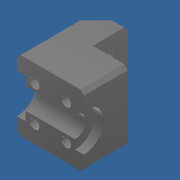
# Autodesk Inventor part: Print_Parts_L
Saved by Autodesk Inventor 2020 (Build 240168000, 168)
## iProperties
Created: 2020-10-05
Part Number: Print_Parts_L
Material: PC/ABS プラスチック
Document SubType Name: Modeling
Designer: kenta iguchi
Density: 0.357273 g/cm^3
Appearance: 滑らか - 黒
Author: kenta iguchi
Autodesk Inventor part; units mm, degrees
ref_plane "YZ Plane" through (0, 0, 0) normal (1, 0, 0) x (0, 1, 0)
ref_plane "XZ Plane" through (0, 0, 0) normal (0, 1, 0) x (-1, 0, 0)
ref_plane "XY Plane" through (0, 0, 0) normal (0, 0, 1) x (1, 0, 0)
sketch "スケッチ1" plane through (0, 0, 0) normal (0, 0, 1) x (1, 0, 0)
  line L0 (-10, -20) -> (10, -20)
  line L1 (10, -20) -> (10, 20)
  line L2 (10, 20) -> (-10, 20)
  line L3 (-10, 20) -> (-10, -20)
  line L4 (-10, -20) -> (10, 20) construction
  line L5 (10, -20) -> (-10, 20) construction
  point P0 (0, 0)
  dimension "d0" = 20
  dimension "d1" = 40
  constraints: 12 end point, 2 midpoint, 2 parallel, 1 horizontal, 1 perpendicular
  measures "d0" distance of L2.end L1.end
  measures "d1" distance of L1.end L0.end
extrude "押し出し1" add sketch "スケッチ1" along normal blind 25
sketch "スケッチ2" plane through (10, -20, 0) normal (1, 0, 0) x (0, 0, -1)
  circle A0 centre (-25, 20) radius 11.1
  line L0 (0, 40) -> (-25, 40) projected
  dimension "d4" = 22.2
  dimension "d7" = 20
  constraints: 1 centre point, 1 vertical alignment
  measures "d4" diameter of A0
  measures "d7" distance from line of L0 A0.centre
extrude "押し出し2" cut sketch "スケッチ2" against normal through all
sketch "スケッチ7" plane through (0, 0, 0) normal (1, 0, 0) x (0, 1, 0)
  arc A0 (-11.1, 25) -> (11.1, 25) centre (0, 25) ccw projected
  line L0 (20, 25) -> (11.1, 25) projected
  line L1 (20, 0) -> (20, 25) projected
  line L2 (20, 0) -> (-20, 0) projected
  line L3 (-20, 0) -> (-20, 25) projected
  line L4 (-11.1, 25) -> (-20, 25) projected
  circle A1 centre (0, 25) radius 6
  arc A2 (-11.1, 25) -> (11.1, 25) centre (0, 25) ccw projected
  line L5 (11.1, 25) -> (-11.1, 25)
  point P0 (0, 0)
  point P1 (-6, 25)
  point P2 (6, 25)
  dimension "d27" = 12
  constraints: 2 end point, 1 centre point, 1 coincident, 1 horizontal
  measures "d27" diameter of A1
extrude "押し出し5" add sketch "スケッチ7" along normal mid plane 10 contours L5 A1 A0
sketch "スケッチ5" plane through (0, 0, 25) normal (0, 0, 1) x (1, 0, 0)
  line L0 (10, 20) -> (-10, 20) projected
  line L1 (-10, -20) -> (10, -20) projected
  point P0 (0, 0)
  point P1 (0, 10)
  point P2 (0, -10)
  dimension "d18" = 10
  dimension "d19" = 10
  measures "d18" distance from line of point (0, 10) L0
  measures "d19" distance from line of point (0, -10) L1
hole "穴1" at (0, 10, 25) at (0, -10, 25) direction (0, 0, -1) diameter 5.3 depth 58
sketch "Sketch9" plane through (-10, -20, 0) normal (-1, 0, 0) x (0, 0, 1)
  arc A0 (25, 31.1) -> (25, 8.9) centre (25, 20) ccw projected
  line L0 (25, 40) -> (25, 31.1) projected
  line L1 (0, 40) -> (25, 40) projected
  line L2 (0, 40) -> (0, 0) projected
  line L3 (0, 0) -> (25, 0) projected
  line L4 (25, 8.9) -> (25, 0) projected
  point P0 (0, 20)
extrude "Extrusion7" add sketch "Sketch9" along normal blind 18
sketch "Sketch10" plane through (0, 0, 0) normal (0, 0, -1) x (-1, 0, 0)
  circle A0 centre (0, 10) radius 2.65 projected
  circle A1 centre (0, -10) radius 2.65 projected
  line L0 (28, -20) -> (-10, -20) projected
  line L1 (28, 20) -> (28, -20) projected
  line L2 (-10, 20) -> (28, 20) projected
  line L3 (-10, -20) -> (-10, 20) projected
  line L4 (-10, -20) -> (-10, -11.1) projected
  line L5 (-10, 20) -> (28, 20) projected
  line L6 (-10, -20) -> (10, -20)
  line L7 (10, -20) -> (10, 20)
  line L8 (10, 20) -> (-10, 20)
  line L9 (-10, 20) -> (-10, -20)
  point P0 (0, 0)
  dimension "d34" = 20
  constraints: 8 end point, 2 parallel, 1 horizontal, 1 perpendicular, 1 point on line
  measures "d34" distance of L8.end L7.end
extrude "Extrusion8" add sketch "Sketch10" along normal blind 20 contours L0 L7 L2 L1
sketch "Sketch11" plane through (-5, 0, 0) normal (-1, 0, 0) x (0, 0, 1)
  line L0 (0, 7.35) -> (25, 7.35) projected
  line L1 (25, -11.1) -> (25, -6) projected
  arc A0 (25, 6) -> (25, -6) centre (25, 0) ccw projected
  line L2 (25, 6) -> (25, 11.1) projected
  arc A1 (25, 11.1) -> (25, -11.1) centre (25, 0) ccw projected
  point P0 (0, 0)
extrude "Extrusion9" add sketch "Sketch11" along normal blind 18
chamfer "Chamfer2" distance 10 angle 45 1 edges at (-28, 0, -20)
sketch "Sketch12" plane through (0, 0, 25) normal (0, 0, 1) x (1, 0, 0)
  line L0 (10, -20) -> (10, -11.1) projected
  circle A0 centre (0, -10) radius 2.65 projected
  line L1 (10, -11.1) -> (5, -11.1) projected
  line L2 (5, -6) -> (5, -11.1) projected
  line L3 (5, -6) -> (-23, -6) projected
  line L4 (-23, -11.1) -> (-23, -6) projected
  line L5 (-23, -11.1) -> (-28, -11.1) projected
  line L6 (-28, -20) -> (-28, -11.1) projected
  line L7 (10, -20) -> (-28, -20) projected
  line L8 (10, -20) -> (10, -11.1) projected
  circle A1 centre (0, 10) radius 2.65 projected
  line L9 (-28, 11.1) -> (-23, 11.1) projected
  line L10 (-23, 6) -> (-23, 11.1) projected
  line L11 (-23, 6) -> (5, 6) projected
  line L12 (5, 11.1) -> (5, 6) projected
  line L13 (5, 11.1) -> (10, 11.1) projected
  line L14 (10, 11.1) -> (10, 20) projected
  line L15 (10, 20) -> (-28, 20) projected
  line L16 (-28, 11.1) -> (-28, 20) projected
  point P0 (0, 0)
  point P1 (-18, -10)
  point P2 (-18, 10)
  dimension "d42" = 28
  constraints: 2 horizontal alignment, 1 vertical alignment
  measures "d42" distance from line of point (-18, -10) L0
hole "Hole2" at (-18, -10, 25) at (-18, 10, 25) direction (0, 0, -1) diameter 5.4 depth 10
chamfer "Chamfer3" distance 2 angle 45 8 edges at (10, -20, 12.5) (10, 20, 12.5) (-28, -20, 7.5) (-28, 20, 7.5) (-23, 20, -15) (-23, -20, -15) (-14, 20, -20) (-14, -20, -20)
sketch "スケッチ13" plane through (-28, -20, 0) normal (-1, 0, 0) x (0, 0, 1)
  line L0 (-20, 38) -> (-10, 38) projected
  line L1 (-20, 38) -> (-20, 2) projected
  line L2 (-10, 2) -> (-20, 2) projected
  line L3 (-10, 2) -> (-10, 38) projected
  line L4 (-9.1716, 0) -> (25, 0) projected
  line L5 (25, 0) -> (25, 2) projected
  line L6 (25, 2) -> (-10, 2) projected
  line L7 (-9.1716, 0) -> (-10, 2) projected
  line L8 (-10, 38) -> (25, 38) projected
  line L9 (25, 38) -> (25, 40) projected
  line L10 (25, 40) -> (-9.1716, 40) projected
  line L11 (-9.1716, 40) -> (-10, 38) projected
  point P0 (0, 20)
  point P1 (-10, 10)
  point P2 (-10, 30)
  dimension "d53" = 10
  dimension "d54" = 10
  constraints: 2 point on line
  measures "d53" distance from line of point (-10, 30) L10
  measures "d54" distance from line of point (-10, 10) L4
hole "穴3" at (-28, -10, -10) at (-28, 10, -10) direction (1, 0, 0) diameter 4.3 end through all counterbore diameter 8 counterbore depth 13
sketch "スケッチ14" plane through (-15, -10, -10) normal (-1, 0, 0) x (0, 0, 1)
  circle A0 centre (0, 0) radius 2.15 projected
  circle A1 centre (0, 20) radius 4 projected
  circle A2 centre (0, 20) radius 2.15 projected
  line L0 (2.15, -2.15) -> (-2.15, -2.15)
  line L1 (-2.15, -2.15) -> (-2.15, 2.15)
  line L2 (-2.15, 2.15) -> (2.15, 2.15)
  line L3 (2.15, 2.15) -> (2.15, -2.15)
  line L4 (2.15, -2.15) -> (-2.15, 2.15) construction
  line L5 (-2.15, -2.15) -> (2.15, 2.15) construction
  line L6 (2.15, 17.85) -> (-2.15, 17.85)
  line L7 (-2.15, 17.85) -> (-2.15, 22.15)
  line L8 (-2.15, 22.15) -> (2.15, 22.15)
  line L9 (2.15, 22.15) -> (2.15, 17.85)
  line L10 (2.15, 17.85) -> (-2.15, 22.15) construction
  line L11 (-2.15, 17.85) -> (2.15, 22.15) construction
  circle A3 centre (0, 20) radius 2.15 projected
  point P0 (10, 10)
  constraints: 24 end point, 4 midpoint, 4 parallel, 3 tangent, 2 horizontal, 2 perpendicular, 1 point on line
extrude "押し出し10" cut sketch "スケッチ14" against normal blind 0.6 contours A0 | L3 L0 A0 | A0 L2 L3 | A0 L1 L2 | L0 L1 A0 | A2 | L9 L6 A2 | A2 L8 L9 | A2 L7 L8 | L6 L7 A2
sketch "スケッチ15" plane through (-15, -10, -10) normal (-1, 0, 0) x (0, 0, 1)
  line L0 (2.15, -2.15) -> (-2.15, -2.15) projected
  line L1 (-2.15, 2.15) -> (2.15, 2.15) projected
  circle A0 centre (0, 0) radius 4 projected
  line L2 (-2.15, -16.7131) -> (2.15, -16.7131)
  line L3 (2.15, -16.7131) -> (2.15, 35.0465)
  line L4 (2.15, 35.0465) -> (-2.15, 35.0465)
  line L5 (-2.15, 35.0465) -> (-2.15, -16.7131)
  line L6 (-2.15, 17.85) -> (-2.15, 22.15) projected
  line L7 (-2.15, 22.15) -> (2.15, 22.15) projected
  line L8 (2.15, 22.15) -> (2.15, 17.85) projected
  line L9 (2.15, 17.85) -> (-2.15, 17.85) projected
  circle A1 centre (0, 20) radius 4 projected
  point P0 (10, 10)
  point P1 (-2.15, -3.3731)
  point P2 (2.15, -3.3731)
  point P3 (-2.15, 3.3731)
  point P4 (2.15, 3.3731)
  point P5 (2.15, 23.3731)
  point P6 (-2.15, 23.3731)
  point P7 (-2.15, 16.6269)
  point P8 (2.15, 16.6269)
  constraints: 8 end point, 2 parallel, 2 vertical alignment, 1 horizontal, 1 perpendicular
extrude "押し出し11" cut sketch "スケッチ15" against normal blind 0.3 contours L3 A0 L5 L0 | L1 L5 A0 L3 | A1 L5 L9 L3 | A1 L3 L7 L5
